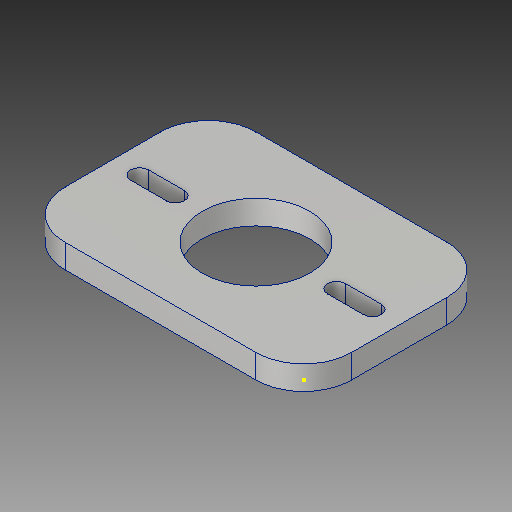
# Autodesk Inventor part: 4461-17-0101 Tensioner Plate
Saved by Autodesk Inventor 2018 (Build 220112000, 112)
## iProperties
Created: 2017-11-02
Part Number: 4461-17-0101 Tensioner Plate
Material: Aluminum 6061
Document SubType Name: Modeling
Designer: s-2513366
Density: 2.7 g/cm^3
Appearance: Aluminum - Flat
Mass: 50.8324 g
Surface Area: 84.0615 cm^2
Volume: 18.8268 cm^3
Author: s-2513366
Autodesk Inventor part; units mm, degrees
ref_plane "YZ Plane" through (0, 0, 0) normal (1, 0, 0) x (0, 1, 0)
ref_plane "XZ Plane" through (0, 0, 0) normal (0, 1, 0) x (-1, 0, 0)
ref_plane "XY Plane" through (0, 0, 0) normal (0, 0, 1) x (1, 0, 0)
sketch "Sketch1" plane through (0, 0, 0) normal (0, 1, 0) x (-1, 0, 0)
  line L0 (0, 0) -> (76.2, 0)
  line L1 (76.2, 0) -> (76.2, -50.8)
  line L2 (76.2, -50.8) -> (0, -50.8)
  line L3 (0, -50.8) -> (0, 0)
  dimension "d0" = 76.2
  dimension "d1" = 50.8
  constraints: 8 end point, 2 parallel, 1 horizontal, 1 perpendicular
  measures "d0" distance of L1.end L2.end
  measures "d1" distance of L0.end L1.end
extrude "Extrusion1" add sketch "Sketch1" along normal blind 6.35
sketch "Sketch2" plane through (0, 6.35, 0) normal (0, 1, 0) x (1, 0, 0)
  line L0 (0, 0) -> (0, 50.8) projected
  line L1 (-76.2, 50.8) -> (-76.2, 0) projected
  line L2 (0, 50.8) -> (-76.2, 0)
  line L3 (-76.2, 0) -> (-76.2, 50.8)
  line L4 (-76.2, 50.8) -> (0, 0)
  circle A0 centre (-38.1, 25.4) radius 14.2875
  dimension "d4" = 28.575
  constraints: 6 end point, 1 centre point, 1 collinear, 1 midpoint
  measures "d4" diameter of A0
hole "Hole1" at (-38.1, 6.35, -25.4) direction (0, -1, 0) diameter 28.575 end through all
sketch "Sketch3" plane through (0, 6.35, 0) normal (0, 1, 0) x (1, 0, 0)
  line L0 (0, 50.8) -> (0, 0) projected
  line L1 (0, 25.4) -> (-23.8125, 25.4)
  circle A0 centre (-38.1, 25.4) radius 14.2875 projected
  line L2 (-52.3875, 25.4) -> (-76.2, 25.4)
  line L3 (-76.2, 0) -> (-76.2, 50.8) projected
  line L4 (-69.0563, 25.4) -> (-59.5312, 25.4) construction
  line L5 (-69.0563, 23.0187) -> (-59.5312, 23.0187)
  line L6 (-59.5312, 27.7812) -> (-69.0563, 27.7812)
  arc A1 (-69.0563, 27.7812) -> (-69.0563, 23.0187) centre (-69.0563, 25.4) ccw
  arc A2 (-59.5312, 23.0187) -> (-59.5312, 27.7812) centre (-59.5312, 25.4) ccw
  line L7 (-16.6688, 25.4) -> (-7.1437, 25.4) construction
  line L8 (-16.6688, 23.0187) -> (-7.1437, 23.0187)
  line L9 (-7.1437, 27.7812) -> (-16.6688, 27.7812)
  arc A3 (-16.6688, 27.7812) -> (-16.6688, 23.0187) centre (-16.6688, 25.4) ccw
  arc A4 (-7.1437, 23.0187) -> (-7.1437, 27.7812) centre (-7.1437, 25.4) ccw
  point P0 (-64.2938, 25.4)
  point P1 (-11.9062, 25.4)
  dimension "d12" = 4.7625
  dimension "d13" = 4.7625
  dimension "d14" = 4.7625
  dimension "d15" = 4.7625
  constraints: 20 end point, 10 point on circle, 8 tangent, 6 midpoint, 4 centre point, 2 parallel, 2 point on line, 1 horizontal
  measures "d12" distance of point (-64.294, 25.4) L4.end
  measures "d13" diameter of A2
  measures "d14" distance of point (-11.906, 25.4) L7.end
  measures "d15" diameter of A4
extrude "Extrusion2" cut sketch "Sketch3" against normal blind 6.35 contours A4 L8 A3 L1 | L1 A3 L9 A4 | A2 L5 A1 L2 | L2 A1 L6 A2
sketch "Sketch4" plane through (0, 6.35, 0) normal (0, 1, 0) x (1, 0, 0)
  point P0 (0, 0)
fillet "Fillet1" radius 12.7 4 edges at (-76.2, 3.175, -50.8) (-76.2, 3.175, 0) (0, 3.175, 0) (0, 3.175, -50.8)
body "Solid1"
